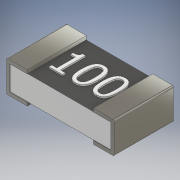
# Autodesk Inventor part: 21-1001
Saved by Autodesk Inventor 2018 (Build 220112000, 112)
## iProperties
Created: 2019-09-21
Part Number: 21-1001
Material: Copper
Document SubType Name: Modeling
Designer: Bradley
Density: 8.94 g/cm^3
Appearance: Smooth - White
Author: Bradley
Autodesk Inventor part; units mm, degrees
ref_plane "YZ Plane" through (0, 0, 0) normal (1, 0, 0) x (0, 1, 0)
ref_plane "XZ Plane" through (0, 0, 0) normal (0, 1, 0) x (-1, 0, 0)
ref_plane "XY Plane" through (0, 0, 0) normal (0, 0, 1) x (1, 0, 0)
sketch "Sketch1" plane through (0, 0, 0) normal (0, 1, 0) x (-1, 0, 0)
  line L0 (0.725, 0.175) -> (-0.725, 0.175)
  line L1 (-0.725, 0.175) -> (-0.725, -0.175)
  line L2 (-0.725, -0.175) -> (0.725, -0.175)
  line L3 (0.725, -0.175) -> (0.725, 0.175)
  line L4 (0.475, 0.175) -> (0.475, 0.225)
  line L5 (0.475, 0.225) -> (0.775, 0.225)
  line L6 (0.775, 0.225) -> (0.775, -0.225)
  line L7 (0.775, -0.225) -> (0.475, -0.225)
  line L8 (0.475, -0.225) -> (0.475, -0.175)
  line L9 (-0.475, 0.175) -> (-0.475, 0.225)
  line L10 (-0.475, 0.225) -> (-0.775, 0.225)
  line L11 (-0.775, 0.225) -> (-0.775, -0.225)
  line L12 (-0.775, -0.225) -> (-0.475, -0.225)
  line L13 (-0.475, -0.175) -> (-0.475, -0.225)
  line L14 (0.475, 0.175) -> (-0.475, 0.175)
  point P0 (0, 0)
  point P1 (0, 0.175)
  point P2 (0.725, 0)
  dimension "d0" = 1.55
  dimension "d1" = 0.05
  dimension "d2" = 0.05
  dimension "d3" = 0.45
  dimension "d4" = 0.3
  constraints: 30 end point, 12 point on line, 7 perpendicular, 3 collinear, 3 midpoint, 2 parallel, 1 horizontal, 1 horizontal alignment, 1 vertical, 1 vertical alignment
  measures "d0" distance between parallel lines of L11 L6
  measures "d1" distance of L7.end L8.end
  measures "d2" distance between parallel lines of L6 L3
  measures "d3" distance of L5.end L6.end
  measures "d4" distance of L6.end L7.end
extrude "Extrusion1" add sketch "Sketch1" along normal mid plane 0.85 contours L0 L4 L5 L6 L7 L8 L2 L3 | L0 L1 L2 L13 L12 L11 L10 L9
extrude "Extrusion2" add sketch "Sketch1" along normal mid plane 0.84 contours L3 L2 L1 L0
sketch "Sketch2" plane through (-0.475, -0.42, 0.175) normal (0, 0, 1) x (1, 0, 0)
  line L0 (0, 0) -> (0, 0.84) projected
  line L1 (0.95, 0) -> (0, 0) projected
  line L2 (0.95, 0) -> (0.95, 0.84) projected
  line L3 (0, 0.84) -> (0.95, 0.84) projected
  line L4 (0, 0.42) -> (0.95, 0.42) construction
  line L5 (0.2805, 0.22) -> (0.0854, 0.22)
  line L6 (0.0854, 0.22) -> (0.0854, 0.2608)
  line L7 (0.0854, 0.2608) -> (0.158, 0.2608)
  line L8 (0.158, 0.2608) -> (0.158, 0.5289)
  line L9 (0.158, 0.5289) -> (0.0854, 0.5289)
  line L10 (0.0854, 0.5289) -> (0.0854, 0.5655)
  spline S0 degree 2 poles (0.0854, 0.5655) (0.1265, 0.5655) (0.1654, 0.5889) (0.168, 0.6213) knots 0 0 0 1 2 2 2
  line L11 (0.168, 0.6213) -> (0.2095, 0.6213)
  line L12 (0.2095, 0.6213) -> (0.2095, 0.2608)
  line L13 (0.2095, 0.2608) -> (0.2805, 0.2608)
  line L14 (0.2805, 0.2608) -> (0.2805, 0.22)
  spline S1 degree 2 poles (0.603, 0.42) (0.603, 0.3124) (0.5405, 0.2116) (0.4753, 0.2116) knots 0 0 0 1 2 2 2
  spline S2 degree 2 poles (0.4753, 0.2116) (0.4092, 0.2116) (0.3473, 0.3143) (0.3473, 0.4197) knots 0 0 0 1 2 2 2
  spline S3 degree 2 poles (0.3473, 0.4197) (0.3473, 0.5279) (0.4098, 0.6281) (0.4753, 0.6281) knots 0 0 0 1 2 2 2
  spline S4 degree 2 poles (0.4753, 0.6281) (0.5411, 0.6281) (0.603, 0.5244) (0.603, 0.42) knots 0 0 0 1 2 2 2
  spline S5 degree 2 poles (0.5343, 0.2981) (0.5421, 0.3179) (0.5486, 0.3788) (0.5486, 0.42) knots 0 0 0 1 2 2 2
  spline S6 degree 2 poles (0.5486, 0.42) (0.5486, 0.4612) (0.5421, 0.5218) (0.534, 0.5422) knots 0 0 0 1 2 2 2
  spline S7 degree 2 poles (0.534, 0.5422) (0.5259, 0.5626) (0.4977, 0.5837) (0.4753, 0.5837) knots 0 0 0 1 2 2 2
  spline S8 degree 2 poles (0.4753, 0.5837) (0.453, 0.5837) (0.4241, 0.5626) (0.4157, 0.5416) knots 0 0 0 1 2 2 2
  spline S9 degree 2 poles (0.4157, 0.5416) (0.4076, 0.5211) (0.4017, 0.4589) (0.4017, 0.4197) knots 0 0 0 1 2 2 2
  spline S10 degree 2 poles (0.4017, 0.4197) (0.4017, 0.3775) (0.4069, 0.3211) (0.4154, 0.2991) knots 0 0 0 1 2 2 2
  spline S11 degree 2 poles (0.4154, 0.2991) (0.4231, 0.2783) (0.452, 0.256) (0.4753, 0.256) knots 0 0 0 1 2 2 2
  spline S12 degree 2 poles (0.4753, 0.256) (0.4974, 0.256) (0.5262, 0.2771) (0.5343, 0.2981) knots 0 0 0 1 2 2 2
  spline S13 degree 2 poles (0.9032, 0.42) (0.9032, 0.3124) (0.8406, 0.2116) (0.7755, 0.2116) knots 0 0 0 1 2 2 2
  spline S14 degree 2 poles (0.7755, 0.2116) (0.7094, 0.2116) (0.6474, 0.3143) (0.6474, 0.4197) knots 0 0 0 1 2 2 2
  spline S15 degree 2 poles (0.6474, 0.4197) (0.6474, 0.5279) (0.71, 0.6281) (0.7755, 0.6281) knots 0 0 0 1 2 2 2
  spline S16 degree 2 poles (0.7755, 0.6281) (0.8413, 0.6281) (0.9032, 0.5244) (0.9032, 0.42) knots 0 0 0 1 2 2 2
  spline S17 degree 2 poles (0.8345, 0.2981) (0.8423, 0.3179) (0.8487, 0.3788) (0.8487, 0.42) knots 0 0 0 1 2 2 2
  spline S18 degree 2 poles (0.8487, 0.42) (0.8487, 0.4612) (0.8423, 0.5218) (0.8342, 0.5422) knots 0 0 0 1 2 2 2
  spline S19 degree 2 poles (0.8342, 0.5422) (0.8261, 0.5626) (0.7979, 0.5837) (0.7755, 0.5837) knots 0 0 0 1 2 2 2
  spline S20 degree 2 poles (0.7755, 0.5837) (0.7531, 0.5837) (0.7243, 0.5626) (0.7158, 0.5416) knots 0 0 0 1 2 2 2
  spline S21 degree 2 poles (0.7158, 0.5416) (0.7077, 0.5211) (0.7019, 0.4589) (0.7019, 0.4197) knots 0 0 0 1 2 2 2
  spline S22 degree 2 poles (0.7019, 0.4197) (0.7019, 0.3775) (0.7071, 0.3211) (0.7155, 0.2991) knots 0 0 0 1 2 2 2
  spline S23 degree 2 poles (0.7155, 0.2991) (0.7233, 0.2783) (0.7521, 0.256) (0.7755, 0.256) knots 0 0 0 1 2 2 2
  spline S24 degree 2 poles (0.7755, 0.256) (0.7975, 0.256) (0.8264, 0.2771) (0.8345, 0.2981) knots 0 0 0 1 2 2 2
  point P0 (0.475, 0.42)
  constraints: 2 end point, 2 midpoint, 1 horizontal
extrude "Extrusion3" add sketch "Sketch2" along normal blind 0.02 contours L5 L6 L7 L8 L9 L10 S0 L11 L12 L13 L14 | S1 S2 S3 S4 | S13 S14 S15 S16
fillet "Fillet1" radius 0.02 4 edges at (-0.775, 0, 0.225) (-0.775, 0, -0.225) (0.775, 0, 0.225) (0.775, 0, -0.225)
equation "\"d2\" = d1"
body "Solid1"
